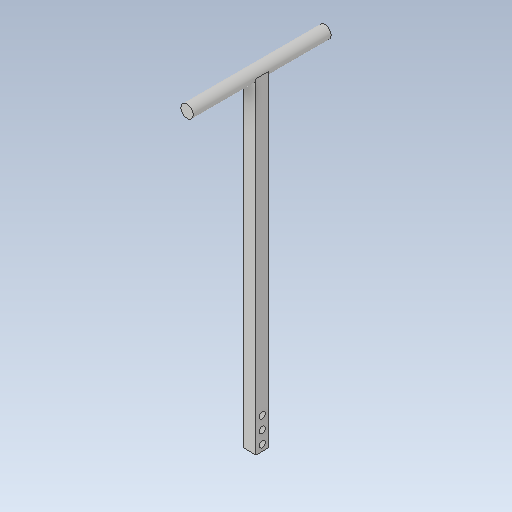
# Autodesk Inventor part: PendulumHanger
Saved by Autodesk Inventor 2020 (Build 240168000, 168)
## iProperties
Created: 2020-04-07
Part Number: PendulumHanger
Material: Generic
Document SubType Name: Modeling
Designer: gman
Density: 1 g/cm^3
Appearance: Default
Mass: 8.61797 g
Surface Area: 57.3815 cm^2
Volume: 8.61797 cm^3
Author: gman
Autodesk Inventor part; units mm, degrees
ref_plane "YZ Plane" through (0, 0, 0) normal (1, 0, 0) x (0, 1, 0)
ref_plane "XZ Plane" through (0, 0, 0) normal (0, 1, 0) x (-1, 0, 0)
ref_plane "XY Plane" through (0, 0, 0) normal (0, 0, 1) x (1, 0, 0)
sketch "Sketch1" plane through (0, 0, 0) normal (0, 0, 1) x (1, 0, 0)
  circle A0 centre (0, 0) radius 3.175
  line L0 (-3.175, 0) -> (-3.175, -165.1)
  line L1 (3.175, 0) -> (3.175, -165.1)
  line L2 (-3.175, -165.1) -> (3.175, -165.1)
  dimension "d0" = 6.35
  dimension "d1" = 165.1
  dimension "d2" = 165.1
  constraints: 6 end point, 2 point on circle, 2 tangent, 2 vertical, 1 centre point, 1 coincident
  measures "d0" diameter of A0
  measures "d1" distance of L0.start L0.end
  measures "d2" distance of L1.start L1.end
extrude "Extrusion1" add sketch "Sketch1" along normal blind 6.35
sketch "Sketch2" plane through (0, 0, 6.35) normal (0, 0, 1) x (1, 0, 0)
  circle A0 centre (0, 0) radius 3.175
  dimension "d5" = 6.35
  constraints: 1 centre point, 1 coincident
  measures "d5" diameter of A0
extrude "Extrusion2" add sketch "Sketch2" along normal blind 31.75
sketch "Sketch3" plane through (0, 0, 0) normal (0, 0, -1) x (-1, 0, 0)
  circle A0 centre (0, 0) radius 3.175
  dimension "d8" = 6.35
  constraints: 1 centre point, 1 coincident
  measures "d8" diameter of A0
extrude "Extrusion3" add sketch "Sketch3" along normal blind 31.75
sketch "Sketch5" plane through (3.175, -165.1, 0) normal (1, 0, 0) x (0, 0, -1)
  circle A0 centre (-3.175, 3.175) radius 1.5875
  circle A1 centre (-3.175, 9.525) radius 1.5875
  circle A2 centre (-3.175, 15.875) radius 1.5875
  line L0 (-6.35, 0) -> (-6.35, 165.1) projected
  line L1 (0, 0) -> (-6.35, 0) projected
  point P0 (0, 165.1)
  dimension "d11" = 3.175
  dimension "d12" = 3.175
  dimension "d13" = 3.175
  dimension "d14" = 3.175
  dimension "d15" = 3.175
  dimension "d16" = 6.35
  dimension "d17" = 6.35
  constraints: 3 centre point, 2 vertical alignment
  measures "d11" diameter of A0
  measures "d12" diameter of A1
  measures "d13" diameter of A2
  measures "d14" distance from line of L0 A0.centre
  measures "d15" distance from line of A0.centre L1
  measures "d16" distance of A0.centre A1.centre
  measures "d17" distance of A1.centre A2.centre
extrude "Extrusion4" cut sketch "Sketch5" against normal blind 12.7
body "Solid1"
